Autodesk Inventor part; units mm, degrees
(part 2 of 2)
  arc A533 (-2.5957, 31.26) -> (-2.7706, 31.3672) centre (-2.7404, 31.2203) ccw
  arc A534 (-2.5957, 31.26) -> (-2.4619, 30.9676) centre (-1.6313, 31.5245) ccw
  arc A535 (-2.4619, 30.9676) -> (-1.9261, 30.727) centre (-2.0011, 31.2769) ccw
  arc A536 (-1.9401, 30.7263) -> (-1.4364, 31.0321) centre (-1.9323, 31.2813) ccw
  arc A537 (-1.4364, 31.0321) -> (-1.3401, 31.339) centre (-2.33, 31.481) ccw
  arc A538 (-1.1799, 31.4673) -> (-1.3401, 31.339) centre (-1.1916, 31.3177) ccw
  line L154 (-0.9299, 31.4643) -> (-1.1799, 31.4673)
  circle A539 centre (0, 0) radius 31.5
  line L155 (-4.9797, 31.0816) -> (-4.7347, 31.1313)
  arc A540 (-4.5534, 31.0354) -> (-4.7347, 31.1313) centre (-4.6953, 30.9866) ccw
  arc A541 (-4.5534, 31.0354) -> (-4.4015, 30.7519) centre (-3.6075, 31.3599) ccw
  arc A542 (-4.4015, 30.7519) -> (-3.8516, 30.5454) centre (-3.961, 31.0896) ccw
  arc A543 (-3.8656, 30.5439) -> (-3.3821, 30.8807) centre (-3.8927, 31.0982) ccw
  arc A544 (-3.3821, 30.8807) -> (-3.3053, 31.193) centre (-4.3021, 31.2726) ccw
  arc A545 (-3.1534, 31.3311) -> (-3.3053, 31.193) centre (-3.1557, 31.1811) ccw
  line L156 (-2.9037, 31.3438) -> (-3.1534, 31.3311)
  circle A546 centre (0, 0) radius 31.5
  line L157 (-6.9215, 30.7076) -> (-6.6801, 30.7726)
  arc A547 (-6.4932, 30.6882) -> (-6.6801, 30.7726) centre (-6.6317, 30.6306) ccw
  arc A548 (-6.4932, 30.6882) -> (-6.3237, 30.4148) centre (-5.5695, 31.0715) ccw
  arc A549 (-6.3237, 30.4148) -> (-5.762, 30.2433) centre (-5.9054, 30.7795) ccw
  arc A550 (-5.7758, 30.2409) -> (-5.3144, 30.6074) centre (-5.8377, 30.7924) ccw
  arc A551 (-5.3144, 30.6074) -> (-5.2574, 30.924) centre (-6.2572, 30.9408) ccw
  arc A552 (-5.1145, 31.0713) -> (-5.2574, 30.924) centre (-5.1074, 30.9214) ccw
  line L158 (-4.8661, 31.0996) -> (-5.1145, 31.0713)
  circle A553 centre (0, 0) radius 31.5
  line L159 (-8.836, 30.2124) -> (-8.5991, 30.2924)
  arc A554 (-8.4073, 30.2199) -> (-8.5991, 30.2924) centre (-8.5419, 30.1538) ccw
  arc A555 (-8.4073, 30.2199) -> (-8.221, 29.9577) centre (-7.5095, 30.6604) ccw
  arc A556 (-8.221, 29.9577) -> (-7.6496, 29.8219) centre (-7.8264, 30.348) ccw
  arc A557 (-7.6633, 29.8185) -> (-7.2258, 30.2133) centre (-7.7596, 30.3651) ccw
  arc A558 (-7.2258, 30.2133) -> (-7.1887, 30.5328) centre (-8.1877, 30.4868) ccw
  arc A559 (-7.0554, 30.6888) -> (-7.1887, 30.5328) centre (-7.0389, 30.5397) ccw
  line L160 (-6.8093, 30.7327) -> (-7.0554, 30.6888)
  circle A560 centre (0, 0) radius 31.5
  line L161 (-10.7156, 29.5979) -> (-10.4842, 29.6927)
  arc A561 (-10.2882, 29.6324) -> (-10.4842, 29.6927) centre (-10.4184, 29.5579) ccw
  arc A562 (-10.2882, 29.6324) -> (-10.0859, 29.3824) centre (-9.4199, 30.1284) ccw
  arc A563 (-10.0859, 29.3824) -> (-9.507, 29.2827) centre (-9.7165, 29.7966) ccw
  arc A564 (-9.5205, 29.2785) -> (-9.1087, 29.7) centre (-9.651, 29.818) ccw
  arc A565 (-9.1087, 29.7) -> (-9.0917, 30.0212) centre (-10.0858, 29.9126) ccw
  arc A566 (-8.9684, 30.1853) -> (-9.0917, 30.0212) centre (-8.9426, 30.0375) ccw
  line L162 (-8.7255, 30.2445) -> (-8.9684, 30.1853)
  circle A567 centre (0, 0) radius 31.5
  line L163 (-12.5529, 28.8667) -> (-12.328, 28.9758)
  arc A568 (-12.1285, 28.9279) -> (-12.328, 28.9758) centre (-12.2538, 28.8454) ccw
  arc A569 (-12.1285, 28.9279) -> (-11.9109, 28.6911) centre (-11.2931, 29.4775) ccw
  arc A570 (-11.9109, 28.6911) -> (-11.327, 28.6279) centre (-11.5683, 29.1277) ccw
  arc A571 (-11.3401, 28.623) -> (-10.9556, 29.0694) centre (-11.5042, 29.1531) ccw
  arc A572 (-10.9556, 29.0694) -> (-10.9588, 29.3911) centre (-11.9441, 29.2203) ccw
  arc A573 (-10.8461, 29.5626) -> (-10.9588, 29.3911) centre (-10.811, 29.4167) ccw
  line L164 (-10.6074, 29.637) -> (-10.8461, 29.5626)
  circle A574 centre (0, 0) radius 31.5
  line L165 (-14.3407, 28.0215) -> (-14.1231, 28.1446)
  arc A575 (-13.921, 28.1093) -> (-14.1231, 28.1446) centre (-14.0409, 28.0191) ccw
  arc A576 (-13.921, 28.1093) -> (-13.6889, 27.8866) centre (-13.1217, 28.7102) ccw
  arc A577 (-13.6889, 27.8866) -> (-13.1022, 27.8602) centre (-13.3744, 28.3439) ccw
  arc A578 (-13.115, 27.8544) -> (-12.7592, 28.3242) centre (-13.312, 28.3732) ccw
  arc A579 (-12.7592, 28.3242) -> (-12.7827, 28.645) centre (-13.7553, 28.4126) ccw
  arc A580 (-12.6809, 28.8232) -> (-12.7827, 28.645) centre (-12.6368, 28.6798) ccw
  line L166 (-12.4474, 28.9124) -> (-12.6809, 28.8232)
  circle A581 centre (0, 0) radius 31.5
  line L167 (-16.0719, 27.0658) -> (-15.8624, 27.2022)
  arc A582 (-15.6585, 27.1797) -> (-15.8624, 27.2022) centre (-15.7725, 27.0822) ccw
  arc A583 (-15.6585, 27.1797) -> (-15.4129, 26.9721) centre (-14.8985, 27.8296) ccw
  arc A584 (-15.4129, 26.9721) -> (-14.8257, 26.9826) centre (-15.1277, 27.4482) ccw
  arc A585 (-14.8381, 26.976) -> (-14.5125, 27.4671) centre (-15.0674, 27.4814) ccw
  arc A586 (-14.5125, 27.4671) -> (-14.5561, 27.7858) centre (-15.5122, 27.4928) ccw
  arc A587 (-14.4657, 27.9701) -> (-14.5561, 27.7858) centre (-14.4127, 27.8298) ccw
  line L168 (-14.2382, 28.0738) -> (-14.4657, 27.9701)
  circle A588 centre (0, 0) radius 31.5
  line L169 (-17.7396, 26.0032) -> (-17.5391, 26.1526)
  arc A589 (-17.3343, 26.1429) -> (-17.5391, 26.1526) centre (-17.4419, 26.0384) ccw
  arc A590 (-17.3343, 26.1429) -> (-17.0761, 25.9511) centre (-16.6166, 26.8392) ccw
  arc A591 (-17.0761, 25.9511) -> (-16.4907, 25.9984) centre (-16.8213, 26.4441) ccw
  arc A592 (-16.5026, 25.991) -> (-16.2086, 26.5017) centre (-16.7632, 26.4811) ccw
  arc A593 (-16.2086, 26.5017) -> (-16.272, 26.817) centre (-17.2079, 26.4646) ccw
  arc A594 (-16.1934, 27.0066) -> (-16.272, 26.817) centre (-16.1317, 26.8699) ccw
  line L170 (-15.9729, 27.1244) -> (-16.1934, 27.0066)
  circle A595 centre (0, 0) radius 31.5
  line L171 (-19.3374, 24.838) -> (-19.1467, 24.9997)
  arc A596 (-18.9416, 25.0029) -> (-19.1467, 24.9997) centre (-19.0424, 24.8918) ccw
  arc A597 (-18.9416, 25.0029) -> (-18.6719, 24.8276) centre (-18.269, 25.7429) ccw
  arc A598 (-18.6719, 24.8276) -> (-18.0906, 24.9117) centre (-18.4486, 25.3357) ccw
  arc A599 (-18.1021, 24.9035) -> (-17.8406, 25.4316) centre (-18.3929, 25.3763) ccw
  arc A600 (-17.8406, 25.4316) -> (-17.9238, 25.7424) centre (-18.8357, 25.3319) ccw
  arc A601 (-17.8572, 25.9365) -> (-17.9238, 25.7424) centre (-17.787, 25.8039) ccw
  line L172 (-17.6446, 26.0679) -> (-17.8572, 25.9365)
  circle A602 centre (0, 0) radius 31.5
  line L173 (-20.8588, 23.5748) -> (-20.6786, 23.7481)
  arc A603 (-20.4742, 23.7642) -> (-20.6786, 23.7481) centre (-20.5678, 23.647) ccw
  arc A604 (-20.4742, 23.7642) -> (-20.194, 23.6062) centre (-19.8494, 24.545) ccw
  arc A605 (-20.194, 23.6062) -> (-19.6191, 23.7266) centre (-20.003, 24.1273) ccw
  arc A606 (-19.6301, 23.7178) -> (-19.4023, 24.2612) centre (-19.95, 24.1713) ccw
  arc A607 (-19.4023, 24.2612) -> (-19.5048, 24.5661) centre (-20.3891, 24.0992) ccw
  arc A608 (-19.4506, 24.764) -> (-19.5048, 24.5661) centre (-19.3722, 24.6362) ccw
  line L174 (-19.2466, 24.9086) -> (-19.4506, 24.764)
  circle A609 centre (0, 0) radius 31.5
  line L175 (-22.2979, 22.2185) -> (-22.129, 22.4028)
  arc A610 (-21.9259, 22.4317) -> (-22.129, 22.4028) centre (-22.012, 22.3089) ccw
  arc A611 (-21.9259, 22.4317) -> (-21.6364, 22.2917) centre (-21.3514, 23.2502) ccw
  arc A612 (-21.6364, 22.2917) -> (-21.0702, 22.4479) centre (-21.4785, 22.8237) ccw
  arc A613 (-21.0806, 22.4384) -> (-20.8874, 22.9951) centre (-21.4283, 22.8709) ccw
  arc A614 (-20.8874, 22.9951) -> (-21.0088, 23.2929) centre (-21.8621, 22.7714) ccw
  arc A615 (-20.9671, 23.4939) -> (-21.0088, 23.2929) centre (-20.8808, 23.3712) ccw
  line L176 (-20.7726, 23.6509) -> (-20.9671, 23.4939)
  circle A616 centre (0, 0) radius 31.5
  line L177 (-23.649, 20.7746) -> (-23.492, 20.9691)
  arc A617 (-23.2912, 21.0107) -> (-23.492, 20.9691) centre (-23.3694, 20.8827) ccw
  arc A618 (-23.2912, 21.0107) -> (-22.9934, 20.8891) centre (-22.7692, 21.8637) ccw
  arc A619 (-22.9934, 20.8891) -> (-22.4381, 21.0806) centre (-22.8693, 21.4301) ccw
  arc A620 (-22.4479, 21.0704) -> (-22.29, 21.6382) centre (-22.8221, 21.4803) ccw
  arc A621 (-22.29, 21.6382) -> (-22.4299, 21.9278) centre (-23.2487, 21.3537) ccw
  arc A622 (-22.4009, 22.131) -> (-22.4299, 21.9278) centre (-22.3071, 22.0139) ccw
  line L178 (-22.2167, 22.2999) -> (-22.4009, 22.131)
  circle A623 centre (0, 0) radius 31.5
  line L179 (-24.9068, 19.2487) -> (-24.7623, 19.4527)
  arc A624 (-24.5645, 19.5068) -> (-24.7623, 19.4527) centre (-24.6345, 19.3741) ccw
  arc A625 (-24.5645, 19.5068) -> (-24.2597, 19.4041) centre (-24.0971, 20.3908) ccw
  arc A626 (-24.2597, 19.4041) -> (-23.7175, 19.6301) centre (-24.1697, 19.9518) ccw
  arc A627 (-23.7266, 19.6193) -> (-23.6047, 20.1958) centre (-24.1258, 20.0049) ccw
  arc A628 (-23.6047, 20.1958) -> (-23.7625, 20.4761) centre (-24.5437, 19.8518) ccw
  arc A629 (-23.7463, 20.6807) -> (-23.7625, 20.4761) centre (-23.6454, 20.5698) ccw
  line L180 (-23.573, 20.8609) -> (-23.7463, 20.6807)
  circle A630 centre (0, 0) radius 31.5
  line L181 (-26.0663, 17.6468) -> (-25.9349, 17.8594)
  arc A631 (-25.7408, 17.9259) -> (-25.9349, 17.8594) centre (-25.8024, 17.7891) ccw
  arc A632 (-25.7408, 17.9259) -> (-25.4302, 17.8426) centre (-25.3299, 18.8375) ccw
  arc A633 (-25.4302, 17.8426) -> (-24.9033, 18.1021) centre (-25.3748, 18.3948) ccw
  arc A634 (-24.9117, 18.0908) -> (-24.8263, 18.6738) centre (-25.3344, 18.4505) ccw
  arc A635 (-24.8263, 18.6738) -> (-25.0014, 18.9437) centre (-25.7417, 18.2715) ccw
  arc A636 (-24.998, 19.1489) -> (-25.0014, 18.9437) centre (-24.8903, 19.0445) ccw
  line L182 (-24.8364, 19.3396) -> (-24.998, 19.1489)
  circle A637 centre (0, 0) radius 31.5
  line L183 (-27.1229, 15.9752) -> (-27.0051, 16.1957)
  arc A638 (-26.8156, 16.2742) -> (-27.0051, 16.1957) centre (-26.8685, 16.1338) ccw
  arc A639 (-26.8156, 16.2742) -> (-26.5004, 16.2106) centre (-26.4627, 17.2099) ccw
  arc A640 (-26.5004, 16.2106) -> (-25.9908, 16.5027) centre (-26.4798, 16.7652) ccw
  arc A641 (-25.9985, 16.4909) -> (-25.9498, 17.0781) centre (-26.4429, 16.8234) ccw
  arc A642 (-25.9498, 17.0781) -> (-26.1415, 17.3364) centre (-26.8382, 16.6191) ccw
  arc A643 (-26.1511, 17.5415) -> (-26.1415, 17.3364) centre (-26.037, 17.4441) ccw
  line L184 (-26.0017, 17.7419) -> (-26.1511, 17.5415)
  circle A644 centre (0, 0) radius 31.5
  line L185 (-28.0725, 14.2406) -> (-27.9688, 14.4681)
  arc A645 (-27.7846, 14.5583) -> (-27.9688, 14.4681) centre (-27.8285, 14.4149) ccw
  arc A646 (-27.7846, 14.5583) -> (-27.4659, 14.5146) centre (-27.4911, 15.5143) ccw
  arc A647 (-27.4659, 14.5146) -> (-26.9757, 14.8381) centre (-27.4802, 15.0694) ccw
  arc A648 (-26.9826, 14.8259) -> (-26.971, 15.415) centre (-27.4471, 15.1298) ccw
  arc A649 (-26.971, 15.415) -> (-27.1785, 15.6608) centre (-27.8288, 14.9011) ccw
  arc A650 (-27.2009, 15.8648) -> (-27.1785, 15.6608) centre (-27.081, 15.7748) ccw
  line L186 (-27.0644, 16.0743) -> (-27.2009, 15.8648)
  circle A651 centre (0, 0) radius 31.5
  line L187 (-28.9113, 12.4499) -> (-28.822, 12.6834)
  arc A652 (-28.6439, 12.785) -> (-28.822, 12.6834) centre (-28.6787, 12.6391) ccw
  arc A653 (-28.6439, 12.785) -> (-28.3231, 12.7614) centre (-28.411, 13.7575) ccw
  arc A654 (-28.3231, 12.7614) -> (-27.8542, 13.115) centre (-28.3722, 13.3142) ccw
  arc A655 (-27.8603, 13.1024) -> (-27.8856, 13.6911) centre (-28.3429, 13.3765) ccw
  arc A656 (-27.8856, 13.6911) -> (-28.1082, 13.9233) centre (-28.7095, 13.1243) ccw
  arc A657 (-28.1434, 14.1255) -> (-28.1082, 13.9233) centre (-28.018, 14.0432) ccw
  line L188 (-28.0204, 14.3432) -> (-28.1434, 14.1255)
  circle A658 centre (0, 0) radius 31.5
  line L189 (-29.636, 10.6099) -> (-29.5615, 10.8486)
  arc A659 (-29.3901, 10.9612) -> (-29.5615, 10.8486) centre (-29.4157, 10.8134) ccw
  arc A660 (-29.3901, 10.9612) -> (-29.0685, 10.9578) centre (-29.2188, 11.9464) ccw
  arc A661 (-29.0685, 10.9578) -> (-28.6227, 11.3402) centre (-29.1522, 11.5064) ccw
  arc A662 (-28.6281, 11.3272) -> (-28.6903, 11.9131) centre (-29.1269, 11.5705) ccw
  arc A663 (-28.6903, 11.9131) -> (-28.927, 12.1309) centre (-29.477, 11.2958) ccw
  arc A664 (-28.9748, 12.3305) -> (-28.927, 12.1309) centre (-28.8445, 12.2562) ccw
  line L190 (-28.8657, 12.5554) -> (-28.9748, 12.3305)
  circle A665 centre (0, 0) radius 31.5
  line L191 (-30.2437, 8.7281) -> (-30.1844, 8.971)
  arc A666 (-30.0204, 9.0941) -> (-30.1844, 8.971) centre (-30.0367, 8.945) ccw
  arc A667 (-30.0204, 9.0941) -> (-29.6992, 9.1109) centre (-29.9113, 10.0882) ccw
  arc A668 (-29.6992, 9.1109) -> (-29.2783, 9.5206) centre (-29.8172, 9.6532) ccw
  arc A669 (-29.2828, 9.5073) -> (-29.3817, 10.0881) centre (-29.7959, 9.7188) ccw
  arc A670 (-29.3817, 10.0881) -> (-29.6316, 10.2907) centre (-30.1281, 9.4226) ccw
  arc A671 (-29.6919, 10.4869) -> (-29.6316, 10.2907) centre (-29.5572, 10.4209) ccw
  line L192 (-29.5971, 10.7182) -> (-29.6919, 10.4869)
  circle A672 centre (0, 0) radius 31.5
  line L193 (-30.732, 6.8119) -> (-30.6881, 7.058)
  arc A673 (-30.5322, 7.1912) -> (-30.6881, 7.058) centre (-30.5391, 7.0414) ccw
  arc A674 (-30.5322, 7.1912) -> (-30.2127, 7.2281) centre (-30.4857, 8.1901) ccw
  arc A675 (-30.2127, 7.2281) -> (-29.8183, 7.6634) centre (-30.3645, 7.7619) ccw
  arc A676 (-29.822, 7.6498) -> (-29.9572, 8.2233) centre (-30.3474, 7.8287) ccw
  arc A677 (-29.9572, 8.2233) -> (-30.2193, 8.4098) centre (-30.6603, 7.5122) ccw
  arc A678 (-30.2918, 8.6018) -> (-30.2193, 8.4098) centre (-30.1532, 8.5444) ccw
  line L194 (-30.2117, 8.8386) -> (-30.2918, 8.6018)
  circle A679 centre (0, 0) radius 31.5
  line L195 (-31.0991, 4.8688) -> (-31.0708, 5.1172)
  arc A680 (-30.9235, 5.2599) -> (-31.0708, 5.1172) centre (-30.9209, 5.1099) ccw
  arc A681 (-30.9235, 5.2599) -> (-30.6069, 5.3168) centre (-30.9398, 6.2598) ccw
  arc A682 (-30.6069, 5.3168) -> (-30.2407, 5.776) centre (-30.792, 5.84) ccw
  arc A683 (-30.2435, 5.7622) -> (-30.4144, 6.3261) centre (-30.7791, 5.9077) ccw
  arc A684 (-30.4144, 6.3261) -> (-30.6877, 6.4957) centre (-31.0715, 5.5722) ccw
  arc A685 (-30.7721, 6.6828) -> (-30.6877, 6.4957) centre (-30.6302, 6.6342) ccw
  line L196 (-30.707, 6.9242) -> (-30.7721, 6.6828)
  circle A686 centre (0, 0) radius 31.5
  line L197 (-31.3435, 2.9064) -> (-31.3308, 3.1561)
  arc A687 (-31.1927, 3.3078) -> (-31.3308, 3.1561) centre (-31.1808, 3.1583) ccw
  arc A688 (-31.1927, 3.3078) -> (-30.8804, 3.3845) centre (-31.2718, 4.3047) ccw
  arc A689 (-30.8804, 3.3845) -> (-30.5437, 3.8657) centre (-31.0979, 3.8951) ccw
  arc A690 (-30.5456, 3.8518) -> (-30.7516, 4.4039) centre (-31.0893, 3.9634) ccw
  arc A691 (-30.7516, 4.4039) -> (-31.035, 4.556) centre (-31.36, 3.6103) ccw
  arc A692 (-31.131, 4.7374) -> (-31.035, 4.556) centre (-30.9863, 4.6978) ccw
  line L198 (-31.0812, 4.9824) -> (-31.131, 4.7374)
  circle A693 centre (0, 0) radius 31.5
  line L199 (-31.4641, 0.9326) -> (-31.4671, 1.1826)
  arc A694 (-31.3389, 1.3427) -> (-31.4671, 1.1826) centre (-31.3176, 1.1942) ccw
  arc A695 (-31.3389, 1.3427) -> (-31.0319, 1.4388) centre (-31.4804, 2.3326) ccw
  arc A696 (-31.0319, 1.4388) -> (-30.7261, 1.9403) centre (-31.2811, 1.9347) ccw
  arc A697 (-30.7272, 1.9262) -> (-30.9675, 2.4643) centre (-31.2768, 2.0035) ccw
  arc A698 (-30.9675, 2.4643) -> (-31.2599, 2.5983) centre (-31.5248, 1.634) ccw
  arc A699 (-31.367, 2.7733) -> (-31.2599, 2.5983) centre (-31.2201, 2.7429) ccw
  line L200 (-31.3327, 3.021) -> (-31.367, 2.7733)
  circle A700 centre (0, 0) radius 31.5
  point P0 (-0.4594, 6.128)
  point P1 (-1.3676, 5.9911)
  point P2 (-2.2453, 5.7203)
  point P3 (-3.0728, 5.3218)
  point P4 (-3.8316, 4.8044)
  point P5 (-4.5049, 4.1797)
  point P6 (-5.0775, 3.4616)
  point P7 (-5.5367, 2.6661)
  point P8 (-5.8722, 1.8112)
  point P9 (-6.0766, 0.9157)
  point P10 (-6.1452, -0.0002)
  point P11 (-6.0765, -0.9161)
  point P12 (-5.8721, -1.8115)
  point P13 (-5.5366, -2.6665)
  point P14 (-5.0773, -3.4619)
  point P15 (-4.5046, -4.1799)
  point P16 (-3.8313, -4.8046)
  point P17 (-3.0724, -5.322)
  point P18 (-2.2449, -5.7205)
  point P19 (-1.3673, -5.9912)
  point P20 (-0.4591, -6.128)
  point P21 (0.4594, -6.128)
  point P22 (1.3676, -5.9911)
  point P23 (2.2453, -5.7203)
  point P24 (3.0728, -5.3218)
  point P25 (3.8316, -4.8044)
  point P26 (4.5049, -4.1797)
  point P27 (5.0775, -3.4616)
  point P28 (5.5367, -2.6661)
  point P29 (5.8722, -1.8112)
  point P30 (6.0766, -0.9157)
  point P31 (6.1452, 0.0002)
  point P32 (6.0765, 0.9161)
  point P33 (5.8721, 1.8115)
  point P34 (5.5366, 2.6665)
  point P35 (5.0773, 3.4619)
  point P36 (4.5046, 4.1799)
  point P37 (3.8313, 4.8046)
  point P38 (3.0724, 5.322)
  point P39 (2.2449, 5.7205)
  point P40 (1.3673, 5.9912)
  point P41 (0.4591, 6.128)
  point P42 (0, 6.5)
  point P43 (-0.1349, 6.5)
  point P44 (-0.9929, 13.25)
  point P45 (-1.7981, 13.8841)
  point P46 (-2.3744, 13.7972)
  point P47 (-2.9567, 12.9541)
  point P48 (-3.8473, 13.461)
  point P49 (-4.4043, 13.2892)
  point P50 (-4.8543, 12.3687)
  point P51 (-5.8106, 12.7372)
  point P52 (-6.3357, 12.4843)
  point P53 (-6.6436, 11.5071)
  point P54 (-7.6441, 11.7289)
  point P55 (-8.1257, 11.4006)
  point P56 (-8.2844, 10.3884)
  point P57 (-9.3068, 10.4586)
  point P58 (-9.7341, 10.0622)
  point P59 (-9.7402, 9.0376)
  point P60 (-10.7616, 8.9547)
  point P61 (-11.1251, 8.499)
  point P62 (-10.9784, 7.485)
  point P63 (-11.9761, 7.2508)
  point P64 (-12.2675, 6.746)
  point P65 (-11.9713, 5.7651)
  point P66 (-12.923, 5.3848)
  point P67 (-13.1359, 4.8423)
  point P68 (-12.6969, 3.9165)
  point P69 (-13.5812, 3.3986)
  point P70 (-13.7109, 2.8304)
  point P71 (-13.1388, 1.9804)
  point P72 (-13.9361, 1.3365)
  point P73 (-13.9796, 0.7552)
  point P74 (-13.2872, 0)
  point P75 (-13.9796, -0.7555)
  point P76 (-13.936, -1.3367)
  point P77 (-13.1388, -1.9803)
  point P78 (-13.7109, -2.8306)
  point P79 (-13.5812, -3.3989)
  point P80 (-12.6969, -3.9164)
  point P81 (-13.1358, -4.8425)
  point P82 (-12.9229, -5.3851)
  point P83 (-11.9714, -5.7651)
  point P84 (-12.2674, -6.7462)
  point P85 (-11.9759, -7.251)
  point P86 (-10.9784, -7.4849)
  point P87 (-11.1249, -8.4992)
  point P88 (-10.7615, -8.9549)
  point P89 (-9.7402, -9.0376)
  point P90 (-9.7339, -10.0624)
  point P91 (-9.3066, -10.4588)
  point P92 (-8.2845, -10.3883)
  point P93 (-8.1255, -11.4007)
  point P94 (-7.6439, -11.7291)
  point P95 (-6.6436, -11.507)
  point P96 (-6.3355, -12.4844)
  point P97 (-5.8104, -12.7373)
  point P98 (-4.8544, -12.3687)
  point P99 (-4.404, -13.2893)
  point P100 (-3.8471, -13.4611)
  point P101 (-2.9567, -12.9541)
  point P102 (-2.3742, -13.7972)
  point P103 (-1.7978, -13.8841)
  point P104 (-0.993, -13.25)
  point P105 (-0.2913, -13.997)
  point P106 (0.2916, -13.997)
  point P107 (0.9929, -13.25)
  point P108 (1.7981, -13.8841)
  point P109 (2.3744, -13.7972)
  point P110 (2.9567, -12.9541)
  point P111 (3.8473, -13.461)
  point P112 (4.4043, -13.2892)
  point P113 (4.8543, -12.3687)
  point P114 (5.8106, -12.7372)
  point P115 (6.3357, -12.4843)
  point P116 (6.6436, -11.5071)
  point P117 (7.6441, -11.7289)
  point P118 (8.1257, -11.4006)
  point P119 (8.2844, -10.3884)
  point P120 (9.3068, -10.4586)
  point P121 (9.7341, -10.0622)
  point P122 (9.7402, -9.0376)
  point P123 (10.7616, -8.9547)
  point P124 (11.1251, -8.499)
  point P125 (10.9784, -7.485)
  point P126 (11.9761, -7.2508)
  point P127 (12.2675, -6.746)
  point P128 (11.9713, -5.7651)
  point P129 (12.923, -5.3848)
  point P130 (13.1359, -4.8423)
  point P131 (12.6969, -3.9165)
  point P132 (13.5812, -3.3986)
  point P133 (13.7109, -2.8304)
  point P134 (13.1388, -1.9804)
  point P135 (13.9361, -1.3365)
  point P136 (13.9796, -0.7552)
  point P137 (13.2872, 0)
  point P138 (13.9796, 0.7555)
  point P139 (13.936, 1.3367)
  point P140 (13.1388, 1.9803)
  point P141 (13.7109, 2.8306)
  point P142 (13.5812, 3.3989)
  point P143 (12.6969, 3.9164)
  point P144 (13.1358, 4.8425)
  point P145 (12.9229, 5.3851)
  point P146 (11.9714, 5.7651)
  point P147 (12.2674, 6.7462)
  point P148 (11.9759, 7.251)
  point P149 (10.9784, 7.4849)
  point P150 (11.1249, 8.4992)
  point P151 (10.7615, 8.9549)
  point P152 (9.7402, 9.0376)
  point P153 (9.7339, 10.0624)
  point P154 (9.3066, 10.4588)
  point P155 (8.2845, 10.3883)
  point P156 (8.1255, 11.4007)
  point P157 (7.6439, 11.7291)
  point P158 (6.6436, 11.507)
  point P159 (6.3355, 12.4844)
  point P160 (5.8104, 12.7373)
  point P161 (4.8544, 12.3687)
  point P162 (4.404, 13.2893)
  point P163 (3.8471, 13.4611)
  point P164 (2.9567, 12.9541)
  point P165 (2.3742, 13.7972)
  point P166 (1.7978, 13.8841)
  point P167 (0.993, 13.25)
  point P168 (0.2913, 13.997)
  point P169 (-0.2916, 13.997)
  point P170 (-2.0002, 7.2284)
  point P171 (10.2069, 7.7653)
  point P172 (9.8417, 8.2232)
  point P173 (8.8822, 8.2419)
  point P174 (8.9355, 9.1998)
  point P175 (8.5062, 9.5982)
  point P176 (7.5546, 9.4736)
  point P177 (7.4646, 10.4289)
  point P178 (6.9806, 10.7588)
  point P179 (6.0582, 10.4938)
  point P180 (5.8268, 11.4249)
  point P181 (5.2992, 11.679)
  point P182 (4.4265, 11.2795)
  point P183 (4.059, 12.1657)
  point P184 (3.4993, 12.3384)
  point P185 (2.696, 11.8133)
  point P186 (2.2004, 12.6348)
  point P187 (1.6213, 12.7221)
  point P188 (0.9052, 12.0831)
  point P189 (0.2927, 12.8217)
  point P190 (-0.293, 12.8217)
  point P191 (-0.9058, 12.0831)
  point P192 (-1.6215, 12.7221)
  point P193 (-2.2007, 12.6348)
  point P194 (-2.6966, 11.8131)
  point P195 (-3.4995, 12.3383)
  point P196 (-4.0592, 12.1657)
  point P197 (-4.4271, 11.2793)
  point P198 (-5.2994, 11.6789)
  point P199 (-5.8271, 11.4248)
  dimension "d142" = 360
  constraints: 1300 point on circle, 700 centre point, 402 end point, 1 coincident, 2701 other
extrude "Wyciągnięcie proste2" add sketch "Szkic3" along normal blind 7.5 contours A1 A2 A3 L2 L199 A694 A695 A696 A697 A698 A699 L200 L197 A687 A688 A689 A690 A691 A692 L198 L195 A680 A681 A682 A683 A684 A685 L196 L193 A673 A674 A675 A676 A677 A678 L194 L191 A666 A667 A668 A669 A670 A671 L192 L189 A659 A660 A661 A662 A663 A664 L190 L187 A652 A653 A654 A655 A656 A657 L188 L185 A645 A646 A647 A648 A649 A650 L186 L183 A638 A639 A640 A641 A642 A643 L184 L181 A631 A632 A633 A634 A635 A636 L182 L179 A624 A625 A626 A627 A628 A629 L180 L177 A617 A618 A619 A620 A621 A622 L178 L175 A610 A611 A612 A613 A614 A615 L176 L173 A603 A604 A605 A606 A607 A608 L174 L171 A596 A597 A598 A599 A600 A601 L172 L169 A589 A590 A591 A592 A593 A594 L170 L167 A582 A583 A584 A585 A586 A587 L168 L165 A575 A576 A577 A578 A579 A580 L166 L163 A568 A569 A570 A571 A572 A573 L164 L161 A561 A562 A563 A564 A565 A566 L162 L159 A554 A555 A556 A557 A558 A559 L160 L157 A547 A548 A549 A550 A551 A552 L158 L155 A540 A541 A542 A543 A544 A545 L156 L153 A533 A534 A535 A536 A537 A538 L154 L151 A526 A527 A528 A529 A530 A531 L152 L149 A519 A520 A521 A522 A523 A524 L150 L147 A512 A513 A514 A515 A516 A517 L148 L145 A505 A506 A507 A508 A509 A510 L146 L143 A498 A499 A500 A501 A502 A503 L144 L141 A491 A492 A493 A494 A495 A496 L142 L139 A484 A485 A486 A487 A488 A489 L140 L137 A477 A478 A479 A480 A481 A482 L138 L135 A470 A471 A472 A473 A474 A475 L136 L133 A463 A464 A465 A466 A467 A468 L134 L131 A456 A457 A458 A459 A460 A461 L132 L129 A449 A450 A451 A452 A453 A454 L130 L127 A442 A443 A444 A445 A446 A447 L128 L125 A435 A436 A437 A438 A439 A440 L126 L123 A428 A429 A430 A431 A432 A433 L124 L121 A421 A422 A423 A424 A425 A426 L122 L119 A414 A415 A416 A417 A418 A419 L120 L117 A407 A408 A409 A410 A411 A412 L118 L115 A400 A401 A402 A403 A404 A405 L116 L113 A393 A394 A395 A396 A397 A398 L114 L111 A386 A387 A388 A389 A390 A391 L112 L109 A379 A380 A381 A382 A383 A384 L110 L107 A372 A373 A374 A375 A376 A377 L108 L105 A365 A366 A367 A368 A369 A370 L106 L103 A358 A359 A360 A361 A362 A363 L104 L101 A351 A352 A353 A354 A355 A356 L102 L99 A344 A345 A346 A347 A348 A349 L100 L97 A337 A338 A339 A340 A341 A342 L98 L95 A330 A331 A332 A333 A334 A335 L96 L93 A323 A324 A325 A326 A327 A328 L94 L91 A316 A317 A318 A319 A320 A321 L92 L89 A309 A310 A311 A312 A313 A314 L90 L87 A302 A303 A304 A305 A306 A307 L88 L85 A295 A296 A297 A298 A299 A300 L86 L83 A288 A289 A290 A291 A292 A293 L84 L81 A281 A282 A283 A284 A285 A286 L82 L79 A274 A275 A276 A277 A278 A279 L80 L77 A267 A268 A269 A270 A271 A272 L78 L75 A260 A261 A262 A263 A264 A265 L76 L73 A253 A254 A255 A256 A257 A258 L74 L71 A246 A247 A248 A249 A250 A251 L72 L69 A239 A240 A241 A242 A243 A244 L70 L67 A232 A233 A234 A235 A236 A237 L68 L65 A225 A226 A227 A228 A229 A230 L66 L63 A218 A219 A220 A221 A222 A223 L64 L61 A211 A212 A213 A214 A215 A216 L62 L59 A204 A205 A206 A207 A208 A209 L60 L57 A197 A198 A199 A200 A201 A202 L58 L55 A190 A191 A192 A193 A194 A195 L56 L53 A183 A184 A185 A186 A187 A188 L54 L51 A176 A177 A178 A179 A180 A181 L52 L49 A169 A170 A171 A172 A173 A174 L50 L47 A162 A163 A164 A165 A166 A167 L48 L45 A155 A156 A157 A158 A159 A160 L46 L43 A148 A149 A150 A151 A152 A153 L44 L41 A141 A142 A143 A144 A145 A146 L42 L39 A134 A135 A136 A137 A138 A139 L40 L37 A127 A128 A129 A130 A131 A132 L38 L35 A120 A121 A122 A123 A124 A125 L36 L33 A113 A114 A115 A116 A117 A118 L34 L31 A106 A107 A108 A109 A110 A111 L32 L29 A99 A100 A101 A102 A103 A104 L30 L27 A92 A93 A94 A95 A96 A97 L28 L25 A85 A86 A87 A88 A89 A90 L26 L23 A78 A79 A80 A81 A82 A83 L24 L21 A71 A72 A73 A74 A75 A76 L22 L19 A64 A65 A66 A67 A68 A69 L20 L17 A57 A58 A59 A60 A61 A62 L18 L15 A50 A51 A52 A53 A54 A55 L16 L13 A43 A44 A45 A46 A47 A48 L14 L11 A36 A37 A38 A39 A40 A41 L12 L9 A29 A30 A31 A32 A33 A34 L10 L7 A22 A23 A24 A25 A26 A27 L8 L5 A15 A16 A17 A18 A19 A20 L6 L3 A8 A9 A10 A11 A12 A13 L4 L1 A4 A6 A5
sketch "Szkic15" plane through (0, 9, 0) normal (0, 1, 0) x (1, 0, 0)
  line L0 (0, 0) -> (-15, 0)
  line L1 (7, 0) -> (15, 0)
  line L2 (-15, -7) -> (-15, 7) construction
  arc A0 (-16, -6) -> (-14, -6) centre (-15, -6) ccw
  arc A1 (-14, 6) -> (-16, 6) centre (-15, 6) ccw
  arc A2 (-14, -3.873) -> (-14, 3.873) centre (-15, 0) ccw
  arc A3 (-16, 3.873) -> (-16, -3.873) centre (-15, 0) ccw
  line L3 (-16, 6) -> (-16, 3.873)
  line L4 (-16, -3.873) -> (-16, -6)
  line L5 (-14, -6) -> (-14, -3.873)
  line L6 (-14, 3.873) -> (-14, 6)
  line L7 (0, 0) -> (15, 0)
  line L8 (15, -7) -> (15, 7) construction
  arc A4 (14, -6) -> (16, -6) centre (15, -6) ccw
  arc A5 (16, 6) -> (14, 6) centre (15, 6) ccw
  arc A6 (16, -3.873) -> (16, 3.873) centre (15, 0) ccw
  arc A7 (14, 3.873) -> (14, -3.873) centre (15, 0) ccw
  line L9 (14, 6) -> (14, 3.873)
  line L10 (14, -3.873) -> (14, -6)
  line L11 (16, -6) -> (16, -3.873)
  line L12 (16, 3.873) -> (16, 6)
  line L13 (-4, 0) -> (-7, 0)
  line L14 (-7, 0) -> (0, 0)
  line L15 (0, 0) -> (7, 0)
  line L16 (-7, 0) -> (7, 0) construction
  arc A8 (-6, 1) -> (-6, -1) centre (-6, 0) ccw
  arc A9 (6, -1) -> (6, 1) centre (6, 0) ccw
  line L17 (-6, -1) -> (-3.873, -1)
  line L18 (3.873, -1) -> (6, -1)
  line L19 (6, 1) -> (3.873, 1)
  line L20 (-3.873, 1) -> (-6, 1)
  arc A10 (-3.873, -1) -> (3.873, -1) centre (0, 0) ccw
  arc A11 (3.873, 1) -> (-3.873, 1) centre (0, 0) ccw
  constraints: 48 end point, 30 point on circle, 24 tangent, 12 centre point, 12 parallel, 8 point on line, 3 coincident, 3 collinear, 3 midpoint, 2 horizontal
extrude "Wyciągnięcie proste3" cut sketch "Szkic15" against normal through all
fillet "Zaokrąglenie1" radius 1 1 edges at (32.5, 0, 0)
sketch "Szkic17" plane through (0, 9, 0) normal (0, 1, 0) x (1, 0, 0)
  point P0 (0, 0)
sketch "Szkic19" plane through (0, 0, 0) normal (0, -1, 0) x (1, 0, 0)
  point P0 (0, 0)
sketch "Szkic21" plane through (0, 0, 0) normal (0, -1, 0) x (1, 0, 0)
  arc A0 (-1, 6.9282) -> (-1, -6.9282) centre (0, 0) ccw projected
  line L0 (0, 0) -> (0, -15)
  circle A1 centre (0, -15) radius 4
  line L1 (-4, -15) -> (-6, -15)
  line L2 (4, -15) -> (6, -15)
  arc A2 (-16, -6) -> (-14, -6) centre (-15, -6) ccw projected
  line L3 (-15, -6) -> (-15, -3) construction
  line L4 (-14, -6) -> (-14, -3)
  line L5 (-16, -3) -> (-16, -6)
  arc A3 (-16, -6) -> (-14, -6) centre (-15, -6) ccw
  arc A4 (-14, -3) -> (-16, -3) centre (-15, -3) ccw
  line L6 (-6, -15) -> (-3, -15) construction
  line L7 (-6, -16) -> (-3, -16)
  line L8 (-3, -14) -> (-6, -14)
  arc A5 (-6, -14) -> (-6, -16) centre (-6, -15) ccw
  arc A6 (-3, -16) -> (-3, -14) centre (-3, -15) ccw
  line L9 (6, -15) -> (3, -15) construction
  line L10 (6, -14) -> (3, -14)
  line L11 (3, -16) -> (6, -16)
  arc A7 (6, -16) -> (6, -14) centre (6, -15) ccw
  arc A8 (3, -14) -> (3, -16) centre (3, -15) ccw
  point P0 (-15, -4.5)
  point P1 (-4.5, -15)
  point P2 (4.5, -15)
  point P3 (-3.873, -16)
  point P4 (3.873, -16)
  point P5 (3.873, -14)
  point P6 (-3.873, -14)
  dimension "d169" = 2
  dimension "d170" = 2
  dimension "d171" = 3
  dimension "d172" = 3
  dimension "d173" = 2
  dimension "d174" = 3
  dimension "d175" = 2
  constraints: 30 end point, 14 point on circle, 12 tangent, 7 centre point, 4 horizontal, 3 midpoint, 3 parallel, 2 vertical, 1 coincident
  measures "d169" distance of L1.start L1.end
  measures "d170" distance of L2.start L2.end
  measures "d171" distance of L3.start L3.end
  measures "d172" distance of L1.end L6.end
  measures "d173" diameter of A6
  measures "d174" distance of L2.end L9.end
  measures "d175" diameter of A8
extrude "Wyciągnięcie proste6" cut sketch "Szkic21" against normal through all contours A1 L11 A8 L10 | A1 L10 A7 L11 | L10 A8 L11 A1 L7 A6 L8 | L7 A5 L8 A1 | A1 L8 A6 L7
sketch "Szkic24" plane through (0, 0, 0) normal (0, -1, 0) x (1, 0, 0)
  line L0 (7, -7) -> (-7, -7)
  line L1 (-7, -7) -> (-7, 7)
  line L2 (-7, 7) -> (7, 7)
  line L3 (7, 7) -> (7, -7)
  line L4 (7, -7) -> (-7, 7) construction
  line L5 (-7, -7) -> (7, 7) construction
  circle A0 centre (0, 0) radius 7
  line L6 (-4.9497, -4.9497) -> (-7, -7)
  line L7 (-4.9497, 4.9497) -> (-7, 7)
  line L8 (7, 7) -> (4.9497, 4.9497)
  line L9 (4.9497, -4.9497) -> (7, -7)
  line L10 (-7, -7) -> (-6.2929, -6.2929)
  line L11 (-7, -7) -> (-3.4645, -3.4645) construction
  line L12 (-6.4697, -7.5303) -> (-2.9341, -3.9948)
  line L13 (-3.9948, -2.9341) -> (-7.5303, -6.4697)
  arc A1 (-7.5303, -6.4697) -> (-6.4697, -7.5303) centre (-7, -7) ccw
  arc A2 (-2.9341, -3.9948) -> (-3.9948, -2.9341) centre (-3.4645, -3.4645) ccw
  line L14 (5.5147, 5.5147) -> (3.4645, 3.4645)
  line L15 (3.4645, 3.4645) -> (4.1716, 4.1716)
  line L16 (3.4645, 3.4645) -> (7, 7) construction
  line L17 (3.9948, 2.9341) -> (7.5303, 6.4697)
  line L18 (6.4697, 7.5303) -> (2.9341, 3.9948)
  arc A3 (2.9341, 3.9948) -> (3.9948, 2.9341) centre (3.4645, 3.4645) ccw
  arc A4 (7.5303, 6.4697) -> (6.4697, 7.5303) centre (7, 7) ccw
  line L19 (-7, 7) -> (-3.4645, 3.4645) construction
  line L20 (-7.5303, 6.4697) -> (-3.9948, 2.9341)
  line L21 (-2.9341, 3.9948) -> (-6.4697, 7.5303)
  arc A5 (-6.4697, 7.5303) -> (-7.5303, 6.4697) centre (-7, 7) ccw
  arc A6 (-3.9948, 2.9341) -> (-2.9341, 3.9948) centre (-3.4645, 3.4645) ccw
  line L22 (5.5147, -5.5147) -> (3.4645, -3.4645)
  line L23 (3.4645, -3.4645) -> (7, -7) construction
  line L24 (2.9341, -3.9948) -> (6.4697, -7.5303)
  line L25 (7.5303, -6.4697) -> (3.9948, -2.9341)
  arc A7 (3.9948, -2.9341) -> (2.9341, -3.9948) centre (3.4645, -3.4645) ccw
  arc A8 (6.4697, -7.5303) -> (7.5303, -6.4697) centre (7, -7) ccw
  point P0 (-5.2322, -5.2322)
  point P1 (5.2322, 5.2322)
  point P2 (-5.2322, 5.2322)
  point P3 (5.2322, -5.2322)
  point P4 (-5.4516, -4.3909)
  point P5 (-4.3909, -5.4516)
  point P6 (4.3909, -5.4516)
  point P7 (5.4516, -4.3909)
  point P8 (5.4516, 4.3909)
  point P9 (4.3909, 5.4516)
  point P10 (-4.3909, 5.4516)
  point P11 (-5.4516, 4.3909)
  dimension "d178" = 14
  dimension "d179" = 14
  dimension "d180" = 1
  dimension "d181" = 5
  dimension "d182" = 1.5
  dimension "d183" = 1
  dimension "d184" = 5
  dimension "d185" = 1.5
  dimension "d186" = 5
  dimension "d187" = 1.5
  dimension "d188" = 5
  dimension "d189" = 1.5
  constraints: 60 end point, 20 point on circle, 16 tangent, 9 centre point, 8 point on line, 6 midpoint, 6 parallel, 2 collinear, 1 coincident, 1 horizontal, 1 perpendicular
  measures "d178" distance of L1.end L2.end
  measures "d179" distance of L0.end L1.end
  measures "d180" distance of L0.end L10.end
  measures "d181" distance of L0.end L11.end
  measures "d182" diameter of A2
  measures "d183" distance of L14.end L15.end
  measures "d184" distance of L14.end L16.end
  measures "d185" diameter of A4
  measures "d186" distance of L1.end L19.end
  measures "d187" diameter of A6
  measures "d188" distance of L23.start L23.end
  measures "d189" diameter of A8
extrude "Wyciągnięcie proste7" cut sketch "Szkic24" against normal through all contours L3 L25 A8 L24 L0 | L9 A0 L25 L3 | L0 L24 A0 L9 | A0 L12 A2 L13 L20 A6 L21 L18 A3 L17 L25 A7 L24 | L24 A7 L25 A0 | L12 A1 L13 L1 L0 | L0 L6 A0 L12 | A0 L13 A2 L12 | L17 A0 L8 L3 | L3 L2 L18 A4 L17 | L17 A3 L18 A0 | L1 L13 A0 L6 | L8 A0 L18 L2 | L20 A5 L21 L2 L1 | L1 L7 A0 L20 | A0 L21 A6 L20 | L21 A0 L7 L2
sketch "Szkic25" plane through (0, 0, 0) normal (0, -1, 0) x (1, 0, 0)
  point P0 (0, 0)
